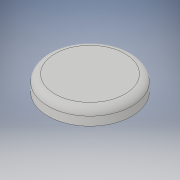
# Autodesk Inventor part: 2016.06.10 ps Hamamatsu PMT Adapter bung cover
Saved by Autodesk Inventor 2017 (Build 210142000, 142)
## iProperties
Created: 2016-06-09
Part Number: 2016.06.10 ps Hamamatsu PMT Adapter bung cover
Material: Generic
Document SubType Name: Modeling
Designer: Darien Morrow
Density: 1 g/cm^3
Appearance: Default
Author: Darien Morrow
Autodesk Inventor part; units mm, degrees
ref_plane "YZ Plane" through (0, 0, 0) normal (1, 0, 0) x (0, 1, 0)
ref_plane "XZ Plane" through (0, 0, 0) normal (0, 1, 0) x (-1, 0, 0)
ref_plane "XY Plane" through (0, 0, 0) normal (0, 0, 1) x (1, 0, 0)
sketch "Sketch1" plane through (0, 0, 0) normal (0, 0, 1) x (1, 0, 0)
  line L0 (0, 0) -> (12.446, 0)
  line L1 (12.446, 0) -> (12.446, 5.588)
  line L2 (12.446, 5.588) -> (0, 5.588)
  line L3 (0, 5.588) -> (0, 0)
  line L4 (0, 5.588) -> (19.05, 5.588)
  line L5 (19.05, 5.588) -> (19.05, 9.525)
  line L6 (15.875, 12.7) -> (0, 12.7)
  line L7 (0, 12.7) -> (0, 5.588)
  arc A0 (19.05, 9.525) -> (15.875, 12.7) centre (15.875, 9.525) ccw
  dimension "d0" = 12.446
  dimension "d1" = 5.588
  dimension "d2" = 19.05
  dimension "d3" = 12.7
  dimension "d4" = 3.175
  constraints: 16 end point, 4 parallel, 2 horizontal, 2 perpendicular, 2 point on circle, 2 tangent, 1 centre point
  measures "d0" distance of L2.end L1.end
  measures "d1" distance between parallel lines of L0 L2
  measures "d2" distance between parallel lines of L5 L7
  measures "d3" distance between parallel lines of L0 L6
  measures "d4" radius of A0
revolve "Revolution1" add sketch "Sketch1" angle 360 about axis through (0, 5.588, 0) along (0, -1, 0)
chamfer "Chamfer1" distance 1.5875 angle 45 1 edges at (-12.446, 0, 0)
body "Solid1"
